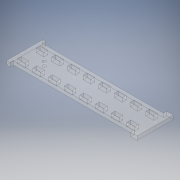
# Autodesk Inventor part: phone_holder_slider
Saved by Autodesk Inventor 2019 (Build 230136000, 136)
## iProperties
Created: 2019-02-17
Part Number: phone_holder_slider
Material: Acrylic, Clear
Document SubType Name: Modeling
Designer: suchanek
Density: 1.19 g/cm^3
Appearance: Transparent - Clear
Author: suchanek
Autodesk Inventor part; units mm, degrees
ref_plane "YZ Plane" through (0, 0, 0) normal (1, 0, 0) x (0, 1, 0)
ref_plane "XZ Plane" through (0, 0, 0) normal (0, 1, 0) x (-1, 0, 0)
ref_plane "XY Plane" through (0, 0, 0) normal (0, 0, 1) x (1, 0, 0)
sketch "Sketch2" plane through (0, 0, 0) normal (0, 1, 0) x (-1, 0, 0)
  line L0 (-100, 22.5) -> (100, 22.5)
  line L1 (100, 22.5) -> (100, -22.5)
  line L2 (100, -22.5) -> (-100, -22.5)
  line L3 (-100, -22.5) -> (-100, 22.5)
  line L4 (-100, 22.5) -> (100, -22.5) construction
  line L5 (100, 22.5) -> (-100, -22.5) construction
  line L6 (100, 22.5) -> (95, 22.5)
  line L7 (95, 22.5) -> (95, 27.5)
  line L8 (95, 27.5) -> (100, 27.5)
  line L9 (100, 27.5) -> (100, 22.5)
  line L10 (100, -22.5) -> (95, -22.5)
  line L11 (95, -22.5) -> (95, -27.5)
  line L12 (95, -27.5) -> (100, -27.5)
  line L13 (100, -27.5) -> (100, -22.5)
  line L14 (-100, -22.5) -> (-90, -22.5)
  line L15 (-90, -22.5) -> (-90, -27.5)
  line L16 (-90, -27.5) -> (-100, -27.5)
  line L17 (-100, -27.5) -> (-100, -22.5)
  line L18 (-100, 22.5) -> (-90, 22.5)
  line L19 (-90, 22.5) -> (-90, 27.5)
  line L20 (-90, 27.5) -> (-100, 27.5)
  line L21 (-100, 27.5) -> (-100, 22.5)
  line L22 (94, 17.5) -> (82, 17.5)
  line L23 (82, 17.5) -> (82, 11.5)
  line L24 (82, 11.5) -> (94, 11.5)
  line L25 (94, 11.5) -> (94, 17.5)
  line L26 (70, 17.5) -> (58, 17.5)
  line L27 (70, 11.5) -> (70, 17.5)
  line L28 (58, 11.5) -> (70, 11.5)
  line L29 (58, 17.5) -> (58, 11.5)
  line L30 (46, 17.5) -> (34, 17.5)
  line L31 (46, 11.5) -> (46, 17.5)
  line L32 (34, 11.5) -> (46, 11.5)
  line L33 (34, 17.5) -> (34, 11.5)
  line L34 (22, 17.5) -> (10, 17.5)
  line L35 (22, 11.5) -> (22, 17.5)
  line L36 (10, 11.5) -> (22, 11.5)
  line L37 (10, 17.5) -> (10, 11.5)
  line L38 (-2, 17.5) -> (-14, 17.5)
  line L39 (-2, 11.5) -> (-2, 17.5)
  line L40 (-14, 11.5) -> (-2, 11.5)
  line L41 (-14, 17.5) -> (-14, 11.5)
  line L42 (-26, 17.5) -> (-38, 17.5)
  line L43 (-26, 11.5) -> (-26, 17.5)
  line L44 (-38, 11.5) -> (-26, 11.5)
  line L45 (-38, 17.5) -> (-38, 11.5)
  line L46 (-50, 17.5) -> (-62, 17.5)
  line L47 (-50, 11.5) -> (-50, 17.5)
  line L48 (-62, 11.5) -> (-50, 11.5)
  line L49 (-62, 17.5) -> (-62, 11.5)
  line L50 (-74, 17.5) -> (-86, 17.5)
  line L51 (-74, 11.5) -> (-74, 17.5)
  line L52 (-86, 11.5) -> (-74, 11.5)
  line L53 (-86, 17.5) -> (-86, 11.5)
  line L54 (94, -11.5) -> (82, -11.5)
  line L55 (94, -17.5) -> (94, -11.5)
  line L56 (82, -17.5) -> (94, -17.5)
  line L57 (82, -11.5) -> (82, -17.5)
  line L58 (70, -11.5) -> (58, -11.5)
  line L59 (70, -17.5) -> (70, -11.5)
  line L60 (58, -17.5) -> (70, -17.5)
  line L61 (58, -11.5) -> (58, -17.5)
  line L62 (46, -11.5) -> (34, -11.5)
  line L63 (46, -17.5) -> (46, -11.5)
  line L64 (34, -17.5) -> (46, -17.5)
  line L65 (34, -11.5) -> (34, -17.5)
  line L66 (22, -11.5) -> (10, -11.5)
  line L67 (22, -17.5) -> (22, -11.5)
  line L68 (10, -17.5) -> (22, -17.5)
  line L69 (10, -11.5) -> (10, -17.5)
  line L70 (-2, -11.5) -> (-14, -11.5)
  line L71 (-2, -17.5) -> (-2, -11.5)
  line L72 (-14, -17.5) -> (-2, -17.5)
  line L73 (-14, -11.5) -> (-14, -17.5)
  line L74 (-26, -11.5) -> (-38, -11.5)
  line L75 (-26, -17.5) -> (-26, -11.5)
  line L76 (-38, -17.5) -> (-26, -17.5)
  line L77 (-38, -11.5) -> (-38, -17.5)
  line L78 (-50, -11.5) -> (-62, -11.5)
  line L79 (-50, -17.5) -> (-50, -11.5)
  line L80 (-62, -17.5) -> (-50, -17.5)
  line L81 (-62, -11.5) -> (-62, -17.5)
  line L82 (-74, -11.5) -> (-86, -11.5)
  line L83 (-74, -17.5) -> (-74, -11.5)
  line L84 (-86, -17.5) -> (-74, -17.5)
  line L85 (-86, -11.5) -> (-86, -17.5)
  circle A0 centre (70, 0) radius 2.5
  point P0 (0, 0)
  point P1 (0, 0)
  dimension "d9" = 45
  dimension "d10" = 200
  dimension "d11" = 5
  dimension "d12" = 5
  dimension "d13" = 5
  dimension "d14" = 5
  dimension "d15" = 10
  dimension "d16" = 5
  dimension "d17" = 10
  dimension "d18" = 5
  dimension "d19" = 12
  dimension "d20" = 6
  dimension "d21" = 6
  dimension "d22" = 5
  dimension "d25" = 24
  dimension "d28" = 29
  dimension "d33" = 5
  dimension "d35" = 25
  constraints: 172 end point, 12 parallel, 7 horizontal, 6 perpendicular, 3 midpoint, 1 centre point, 1 horizontal alignment, 1 vertical, 120 other
  measures "d9" distance of L0.end L1.end
  measures "d10" distance of L1.end L2.end
  measures "d11" distance of L7.end L8.end
  measures "d12" distance of L6.end L7.end
  measures "d13" distance of L12.end L11.end
  measures "d14" distance of L11.end L10.end
  measures "d15" distance of L15.end L16.end
  measures "d16" distance of L14.end L15.end
  measures "d17" distance of L20.end L19.end
  measures "d18" distance of L19.end L18.end
  measures "d19" distance of L24.end L23.end
  measures "d20" distance of L23.end L22.end
  measures "d21" distance between parallel lines of L1 L25
  measures "d22" distance from line of L6.end L22
  measures "d25" distance of L22.start L26.start
  measures "d28" distance of L22.start L54.start
  measures "d33" diameter of A0
  measures "d35" distance from line of A0.centre L11
extrude "Extrusion2" add sketch "Sketch2" along normal blind 6
body "Solid2"
